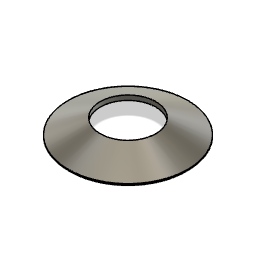
cap v1 (Autodesk Fusion 360 design; units mm, degrees)
Autodesk Fusion 360 part; units mm, degrees
sketch "Sketch1" plane through (0, 0, 0) normal (0, 0, 1) x (1, 0, 0)
  line L0 (-20, 12) -> (-50, -2)
  line L1 (-56, 0) -> (-56, -2)
  line L2 (-56, -2) -> (-54.3535, -2)
  line L3 (-54.3535, -2) -> (-54.3535, -1.995)
  line L4 (-54.3535, -1.995) -> (-27, 10.7699)
  line L5 (-27, 10.7699) -> (-27, 15.3393)
  line L6 (-27, 15.3393) -> (-58, 0.8726)
  line L7 (-58, 0.8726) -> (-58, 0)
  line L8 (-58, 0) -> (-56, 0)
  line L9 (0, 11) -> (0, -10) construction
  dimension "d71" = 58
  dimension "d72" = 56
  dimension "d73" = 2
  dimension "d74" = 27
  constraint vertical L1
  constraint perpendicular L1 L2
  constraint perpendicular L2 L3
  constraint parallel L3 L5
  constraint parallel L1 L7
  constraint perpendicular L1 L8
  constraint vertical L9
  constraint parallel L0 L4
  constraint parallel L4 L6
  measures "d71" distance of L7.end L9
  measures "d72" distance of L1 L9
  measures "d73" distance of L1.end L1.start
  measures "d74" distance of L5 L9
revolve "Revolve1" add sketch "Sketch1" angle 360 about axis through (0, 11, 0) along (0, -1, 0)
named bodies: "cap"
